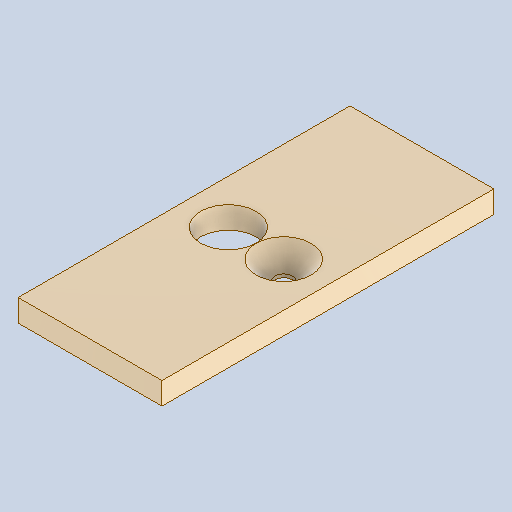
# Autodesk Inventor part: LagerHO
Saved by Autodesk Inventor 2025 (Build 290162010, 162A)
## iProperties
Created: 2024-11-12
Part Number: LagerHO
Material: Polyethylen, hohe Dichte, Gleitfläche
Document SubType Name: Modeling
Designer: Admin
Density: 0.952 g/cm^3
Appearance: Glatt - Eierschale(1)
Author: Admin
Autodesk Inventor part; units mm, degrees
ref_plane "YZ Plane" through (0, 0, 0) normal (1, 0, 0) x (0, 1, 0)
ref_plane "XZ Plane" through (0, 0, 0) normal (0, 1, 0) x (-1, 0, 0)
ref_plane "XY Plane" through (0, 0, 0) normal (0, 0, 1) x (1, 0, 0)
sketch "Skizze1" plane through (0, 0, 0) normal (0, 0, 1) x (1, 0, 0)
  circle A0 centre (6, 15) radius 2.5 projected
  circle A1 centre (11, 15) radius 0.7835 projected
  line L0 (0, 0) -> (15, 0) projected
  line L1 (15, 0) -> (15, 30) projected
  line L2 (0, 30) -> (15, 30) projected
  line L3 (0, 0) -> (0, 30) projected
  line L4 (2, 0) -> (2, 30) projected
extrude "Extrusion1" add sketch "Skizze1" along normal blind 2 contours L4 L2 L1 L0
chamfer "Fasen1" distance 1.7 angle 45 1 edges at (10.2165, 15, 2)
